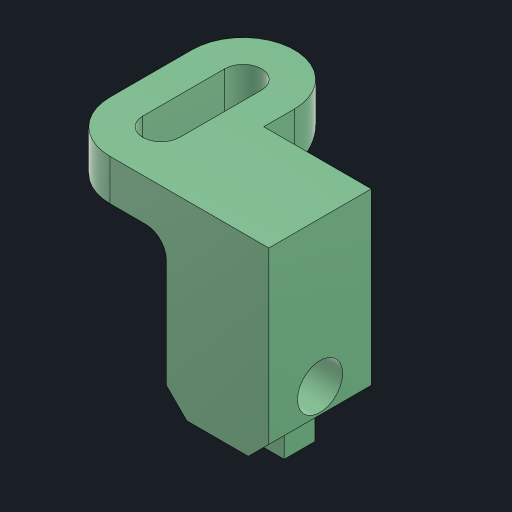
# Autodesk Inventor part: om_Drop_10g_L
Saved by Autodesk Inventor 2023 (Build 270158000, 158)
## iProperties
Created: 2022-06-20
Part Number: om_Drop_10g_L
Material: ABS プラスチック
Document SubType Name: Modeling
Designer: legot
Density: 1.06 g/cm^3
Appearance: 滑らか - 白
Author: legot
Autodesk Inventor part; units mm, degrees
ref_plane "YZ Plane" through (0, 0, 0) normal (1, 0, 0) x (0, 1, 0)
ref_plane "XZ Plane" through (0, 0, 0) normal (0, 1, 0) x (-1, 0, 0)
sketch "スケッチ1" plane through (0, 0, 0) normal (0, 1, 0) x (-1, 0, 0)
  arc A0 (0.9, 0) -> (-0.9, 0) centre (0, 0) ccw
  arc A1 (-0.9, -4) -> (0.9, -4) centre (0, -4) ccw
  line L0 (0, 0) -> (0, -4) construction
  line L1 (-0.9, -4) -> (-0.9, 0)
  line L2 (0.9, -4) -> (0.9, 0)
  arc A2 (-2.5, -4) -> (2.5, -4) centre (0, -4) ccw
  line L3 (-2.5, -4) -> (-2.5, 0)
  arc A3 (2.5, 0) -> (-2.5, 0) centre (0, 0) ccw
  line L4 (2.5, 0) -> (2.5, -4)
  line L5 (-2.5, -2.5) -> (-7.75, -2.5)
  line L6 (-7.75, -2.5) -> (-7.75, 2.5)
  line L7 (-7.75, 2.5) -> (-2.75, 2.5)
  line L8 (-2.75, -2.5) -> (-7.75, -2.5)
  line L9 (-7.75, -2.5) -> (-7.75, 2.5)
  line L10 (-7.75, 2.5) -> (-2.75, 2.5)
  line L11 (-2.75, 2.5) -> (-2.75, -2.5)
  line L12 (-2.75, 2.5) -> (0, 2.5)
  point P0 (-5.25, -2.5)
  point P1 (-3.4, 2.5)
  point P2 (0, 2.5)
  dimension "d0" = 1.8
  dimension "d1" = 4
  dimension "d2" = 1.6
  dimension "d40" = 5
  dimension "d41" = 5.25
  dimension "d42" = 5
  constraints: 26 end point, 10 point on circle, 5 tangent, 4 centre point, 4 parallel, 2 horizontal, 2 perpendicular, 2 point on line, 1 coincident, 1 equal radius, 1 midpoint, 1 vertical, 1 vertical alignment, 3 other
  measures "d0" diameter of A0
  measures "d1" distance of L0.start L0.end
  measures "d2" distance between parallel lines of L3 L1
  measures "d40" distance of L5.end L6.end
  measures "d41" distance from line of L0 point (-5.25, -2.5)
  measures "d42" distance between parallel lines of L9 L11
extrude "押し出し1" add sketch "スケッチ1" along normal blind 2
extrude "押し出し4" add sketch "スケッチ1" against normal blind 7.3 contours L5 L6 L7 L11
sketch "スケッチ6" plane through (7.75, 2, 2.5) normal (1, 0, 0) x (0, 0, -1)
  line L0 (5, -9.3) -> (0, -9.3) projected
  point P0 (2.5, -2)
  point P1 (2.5, -7.1)
  point P2 (2.5, -9.3)
  dimension "d43" = 2.2
  constraints: 1 midpoint, 1 vertical alignment
  measures "d43" distance from line of L0 point (2.5, -7.1)
hole "穴3" at (7.75, -5.1, 0) direction (-1, 0, 0) diameter 2.2 end through all
fillet "フィレット3" radius 1 1 edges at (2.75, 0, 0)
ref_plane "作業平面2" through (0, 0, 0) normal (1, 0, 0) x (0, 0, -1)
chamfer "面取り1" distance 1 angle 45 2 edges at (2.75, -7.3, 0) (7.75, -7.3, 0)
sketch "スケッチ7" plane through (0, -7.3, 0) normal (0, -1, 0) x (1, 0, 0)
  line L0 (6.75, 2.5) -> (6.75, -2.5) projected
  line L1 (3.75, -2.5) -> (3.75, 2.5) projected
  line L2 (6.75, 0.75) -> (3.75, 0.75)
  line L3 (3.75, 0.75) -> (3.75, -0.75)
  line L4 (3.75, -0.75) -> (6.75, -0.75)
  line L5 (6.75, -0.75) -> (6.75, 0.75)
  point P0 (0, 0)
  point P1 (6.75, 0)
  point P2 (6.75, 0.75)
  point P3 (3.75, 0.75)
  dimension "d55" = 1.5
  constraints: 8 end point, 2 midpoint, 2 parallel, 2 point on line, 1 horizontal, 1 perpendicular
  measures "d55" distance between parallel lines of L2 L4
extrude "押し出し5" add sketch "スケッチ7" along normal blind 1
